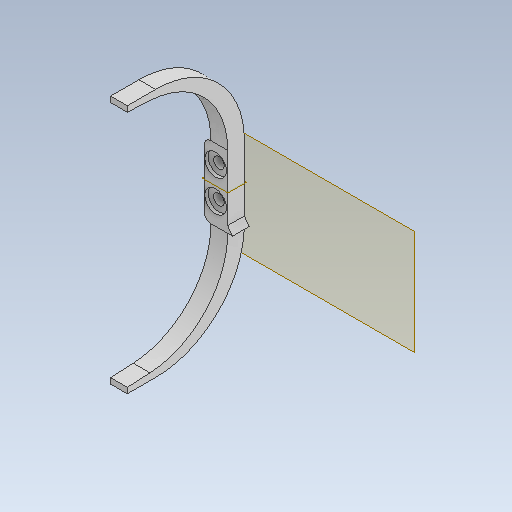
# Autodesk Inventor part: leg
Saved by Autodesk Inventor 2020 (Build 240168000, 168)
## iProperties
Created: 2019-05-07
Part Number: leg
Material: Generic
Document SubType Name: Modeling
Designer: erwin
Density: 1 g/cm^3
Appearance: Default
Author: erwin
Autodesk Inventor part; units mm, degrees
ref_plane "YZ Plane" through (0, 0, 0) normal (1, 0, 0) x (0, 1, 0)
ref_plane "XZ Plane" through (0, 0, 0) normal (0, 1, 0) x (-1, 0, 0)
ref_plane "XY Plane" through (0, 0, 0) normal (0, 0, 1) x (1, 0, 0)
ref_plane "Work Plane1" through (0, 0.5, 0) normal (0, 0, 1) x (1, 0, 0)
sketch "Sketch1" plane through (0, 0.5, 0) normal (0, 0, 1) x (1, 0, 0)
  arc A0 (-25.85, 13.75) -> (-27.85, 11.75) centre (-25.85, 11.75) ccw
  line L0 (-27.85, 11.75) -> (-27.85, -5.75)
  arc A1 (-27.85, -5.75) -> (-25.85, -7.75) centre (-25.85, -5.75) ccw
  line L1 (-25.85, -7.75) -> (-19.4, -7.75)
  arc A2 (-17.4, -9.75) -> (-19.4, -7.75) centre (-19.4, -9.75) ccw
  line L2 (-17.4, -9.75) -> (-17.4, -12.466667)
  arc A3 (-17.4, -12.466667) -> (-15.4, -14.466667) centre (-15.4, -12.466667) ccw
  line L3 (-15.4, -14.466667) -> (1.1, -14.466667)
  arc A4 (1.1, -14.466667) -> (3.1, -12.466667) centre (1.1, -12.466667) ccw
  line L4 (3.1, -12.466667) -> (3.1, -9.75)
  arc A5 (5.1, -7.75) -> (3.1, -9.75) centre (5.1, -9.75) ccw
  line L5 (5.1, -7.75) -> (24.95, -7.75)
  arc A6 (24.95, -7.75) -> (26.95, -5.75) centre (24.95, -5.75) ccw
  line L6 (26.95, -5.75) -> (26.95, 11.941667)
  arc A7 (26.95, 11.941667) -> (24.95, 13.941667) centre (24.95, 11.941667) ccw
  line L7 (24.95, 13.941667) -> (19.95, 13.941667)
  line L8 (19.95, 13.941667) -> (19.95, -5.75)
  line L9 (19.95, -5.75) -> (1.6, -5.75)
  line L10 (1.6, -5.75) -> (1.1, -12.466667)
  line L11 (1.1, -12.466667) -> (-13.9, -12.75)
  line L12 (-15.4, -12.75) -> (-15.4, -5.75)
  line L13 (-15.4, -5.75) -> (-20.85, -5.75)
  line L14 (-20.85, -5.75) -> (-20.85, 13.75)
  line L15 (-20.85, 13.75) -> (-25.85, 13.75)
  circle A8 centre (23.55, -1.25) radius 1.25
  circle A9 centre (-24.45, -1.25) radius 1.25
  circle A10 centre (-24.45, 8.25) radius 1.25
  circle A11 centre (23.55, 8.25) radius 1.25
  line L16 (-20.4, -5.75) -> (-20.4, -7.75)
  line L17 (-13.9, -12.75) -> (-15.4, -12.75)
  point P0 (0, -0.5)
  constraints: 2 end point, 1 vertical
sketch "Sketch1 outline for Extrusion1" plane through (0, 0.5, 0) normal (0, 0, 1) x (1, 0, 0)
  line L0 (-20.85, -5.75) -> (-20.85, 13.75)
  line L1 (-19.4, -7.75) -> (-20.85, -5.75)
  line L2 (-20.85, 13.75) -> (-25.85, 13.75)
  line L3 (-25.85, -7.75) -> (-19.4, -7.75)
  arc A0 (-25.85, 13.75) -> (-27.85, 11.75) centre (-25.85, 11.75) ccw
  arc A1 (-27.85, -5.75) -> (-25.85, -7.75) centre (-25.85, -5.75) ccw
  line L4 (-27.85, 11.75) -> (-27.85, -5.75)
  circle A2 centre (-24.45, -1.25) radius 1.25
  circle A3 centre (-24.45, 8.25) radius 1.25
extrude "Extrusion1" add sketch "Sketch1 outline for Extrusion1" along normal blind 5
ref_plane "Work Plane2" through (-25.85, 3.5, 0) normal (0, -1, 0) x (1, 0, 0)
sketch "Sketch3" plane through (-20.85, -7.25, 0) normal (1, 0, 0) x (0, 0, -1)
  line L0 (0, 19.5) -> (-5, 19.5)
  line L1 (0, 21.5) -> (-5, 21.5)
  line L2 (0, 21.5) -> (0, 19.5)
  arc A0 (0, 21.5) -> (-26.539944, 48.039944) centre (-26.539944, 21.5) ccw
  line L3 (-26.539944, 48.039944) -> (-35, 48.039944)
  line L4 (-35, 48.039944) -> (-35, 46.366043)
  line L5 (-35, 46.366043) -> (-28.232934, 46.005114)
  arc A1 (-5, 21.5) -> (-28.232934, 46.005114) centre (-29.539944, 21.5) ccw
  line L6 (-5, 2) -> (-5, 21.5)
  line L7 (0, 2) -> (0, 21.5)
  point P0 (0, 7.25)
  point P1 (-5, 0)
  point P2 (0, 0)
  dimension "d9" = 3
  dimension "d12" = 35
  constraints: 6 end point, 4 point on circle, 4 tangent, 2 centre point, 1 perpendicular, 1 vertical
  measures "d9" distance of A0.centre A1.centre
  measures "d12" distance between parallel lines of L2 L4
extrude "Extrusion2" add sketch "Sketch3" against normal blind 5 contours L1 A1 L5 L4 L3 A0
sketch "Sketch2" plane through (0, 0.5, 5) normal (0, 0, 1) x (1, 0, 0)
  circle A0 centre (-24.45, -1.25) radius 1.25 projected
  circle A1 centre (-24.45, 8.25) radius 1.25 projected
  point P0 (0, -0.5)
  constraints: 2 coincident
hole "Hole1" at (-24.45, -0.75, 5) at (-24.45, 8.75, 5) direction (0, 0, -1) diameter 3.2 end through all counterbore diameter 6.5 counterbore depth 1
mirror "Mirror1" about plane through (-25.85, 3.5, 0) normal (0, -1, 0) of "Extrusion2"
body "Solid1"
